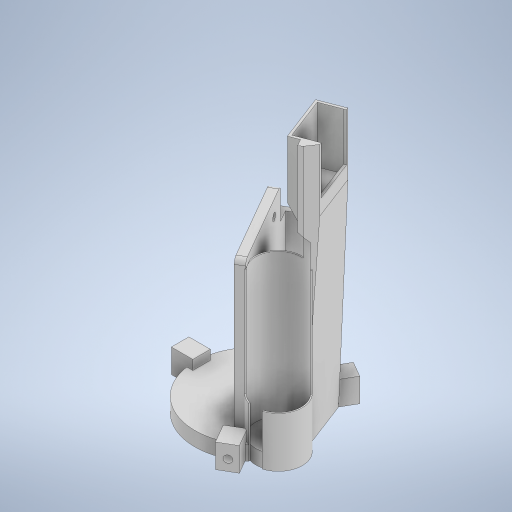
# Autodesk Inventor part: Electronic casing
Saved by Autodesk Inventor 2024 (Build 280153000, 153)
## iProperties
Created: 2024-03-27
Part Number: Electronic casing
Material: Generic
Document SubType Name: Modeling
Designer: auror
Density: 1 g/cm^3
Appearance: Default
Author: auror
Autodesk Inventor part; units mm, degrees
ref_plane "YZ Plane" through (0, 0, 0) normal (1, 0, 0) x (0, 1, 0)
ref_plane "XZ Plane" through (0, 0, 0) normal (0, 1, 0) x (-1, 0, 0)
ref_plane "XY Plane" through (0, 0, 0) normal (0, 0, 1) x (1, 0, 0)
sketch "Sketch9" plane through (0, 0, 0) normal (0, 1, 0) x (-1, 0, 0)
  line L0 (37.6236, 0) -> (-39.3749, 0) construction
  line L1 (0, 0) -> (-26.8726, 46.5447) construction
  line L2 (0, 0) -> (-26.275, -45.5096) construction
  line L3 (31.2294, 3.6686) -> (31.2294, -3.6686)
  line L4 (31.2294, 3.6686) -> (24.7294, 3.6686)
  line L5 (31.2294, -3.6686) -> (24.7294, -3.6686)
  line L6 (0, 0) -> (-18.4784, 42.9064) construction
  line L7 (0, 0) -> (-25.1787, 33.7798) construction
  line L8 (0, 0) -> (31.2294, 3.6686) construction
  line L9 (-12.4376, 28.8797) -> (-18.7918, 25.2111)
  line L10 (-12.4376, 28.8797) -> (-9.1876, 23.2506)
  line L11 (-18.7918, 25.2111) -> (-15.5418, 19.582)
  line L12 (0, 0) -> (-18.2948, -42.48) construction
  line L13 (-18.2948, -42.48) -> (0, 0) construction
  line L14 (0, 0) -> (-26.6993, -35.8199) construction
  line L15 (-18.7918, -25.2111) -> (-12.4376, -28.8797)
  line L16 (-18.7918, -25.2111) -> (-15.5418, -19.582)
  line L17 (-12.4376, -28.8797) -> (-9.1876, -23.2506)
  arc A0 (-15.5418, 19.582) -> (-15.5418, -19.582) centre (0, 0) ccw
  arc A1 (-9.1876, -23.2506) -> (24.7294, -3.6686) centre (0, 0) ccw
  arc A2 (24.7294, 3.6686) -> (-9.1876, 23.2506) centre (0, 0) ccw
  line L18 (0, 0) -> (31.2294, -3.6686) construction
  dimension "d131" = 120
  dimension "d132" = 120
  dimension "d136" = 6.7
  dimension "d137" = 6.7
  dimension "d139" = 6.7
  dimension "d140" = 6.7
  dimension "d220" = 6.5
  dimension "d221" = 6.5
  dimension "d222" = 25
  dimension "d223" = 25
  dimension "d224" = 25
  dimension "d225" = 6.5
  dimension "d227" = 6.5
  dimension "d228" = 6.5
  dimension "d236" = 6.7
  dimension "d237" = 6.7
  constraints: 38 end point, 6 point on circle, 4 perpendicular, 4 point on line, 3 centre point, 3 horizontal, 2 coincident, 1 vertical
  measures "d131" angle of L2 L0
  measures "d132" angle of L1 L0
  measures "d136" angle of L1 L6
  measures "d137" angle of L7 L1
  measures "d139" angle of L2 L12
  measures "d140" angle of L2 L14
  measures "d220" distance of L15.end L17.end
  measures "d221" distance of L9.end L11.end
  measures "d222" radius of A0
  measures "d223" radius of A1
  measures "d224" radius of A2
  measures "d225" distance of L3.end L5.end
  measures "d227" distance of L9.start L10.end
  measures "d228" distance of L15.start L16.end
  measures "d236" angle of L0 L8
  measures "d237" angle of L18 L0
extrude "Extrusion4" add sketch "Sketch9" along normal blind 6
sketch "Sketch10" plane through (18.7918, 0, 25.2111) normal (0.5, 0, 0.8660254) x (0.8660254, 0, -0.5)
  line L0 (0, 0) -> (0, 6) projected
  line L1 (-7.3372, 0) -> (0, 0) projected
  point P0 (-3.6686, 0)
  point P1 (-3.5, 4.5)
  point P2 (0, 3)
  dimension "d143" = 3.5
  dimension "d144" = 4.5
  constraints: 1 midpoint
  measures "d143" horizontal distance of point (0, 3) point (-3.5, 4.5)
  measures "d144" distance from line of L1 point (-3.5, 4.5)
hole "Hole5" at (15.7607, 4.5, 26.9611) direction (-0.5, 0, -0.8660254) diameter 3 depth 8 tip angle 118 counterbore diameter 4 counterbore depth 0
sketch "Sketch11" plane through (12.4376, 0, -28.8797) normal (0.5, 0, -0.8660254) x (-0.8660254, 0, -0.5)
  line L0 (-7.3372, 0) -> (0, 0) projected
  point P0 (-3.6686, 0)
  point P1 (-3.5001, 4.5)
  dimension "d152" = 4.5
  measures "d152" distance from line of L0 point (-3.5, 4.5)
hole "Hole6" at (15.4688, 4.5, -27.1297) direction (-0.5, 0, 0.8660254) diameter 3 depth 8 tip angle 118 counterbore diameter 4 counterbore depth 0
sketch "Sketch12" plane through (-31.2294, 0, -3.6686) normal (-1, 0, 0) x (0, 0, 1)
  line L0 (0, 0) -> (7.3372, 0) projected
  point P0 (3.6686, 0)
  point P1 (3.5, 4.5)
  dimension "d160" = 4.5
  measures "d160" distance from line of L0 point (3.5, 4.5)
hole "Hole7" at (-31.2294, 4.5, -0.1686) direction (1, 0, 0) diameter 3 depth 8 tip angle 118 counterbore diameter 4 counterbore depth 0
sketch "Sketch13" plane through (0, 6, 0) normal (0, 1, 0) x (1, 0, 0)
  line L0 (0, -31.2314) -> (0, 39.2316) construction
  line L1 (11.4285, -21.7947) -> (-13.356, 21.1333) construction
  arc A0 (9.1876, 23.2506) -> (-24.7294, 3.6686) centre (0, 0) ccw construction
  line L2 (8.9539, -17.5087) -> (11.985, -15.7587)
  line L3 (8.9539, -17.5087) -> (-11.0461, 17.1324)
  line L4 (-11.0461, 17.1324) -> (-8.015, 18.8824)
  line L5 (-8.015, 18.8824) -> (11.985, -15.7587)
  dimension "d168" = -30
  dimension "d169" = 1
  dimension "d176" = 40
  dimension "d178" = 3.5
  dimension "d238" = 3.5
  constraints: 12 end point, 2 perpendicular, 2 point on line, 1 collinear, 1 point on circle, 1 vertical
  measures "d168" angle of L0 L1
  measures "d169" distance from line of A0.centre L1
  measures "d176" distance of L3.end L2.start
  measures "d178" distance of L2.start L2.end
  measures "d238" distance of L3.end L4.end
extrude "Extrusion5" add sketch "Sketch13" along normal blind 63
sketch "Sketch14" plane through (0, 6, 0) normal (0, 1, 0) x (1, 0, 0)
  line L0 (11.985, -15.7587) -> (-8.015, 18.8824) projected
  line L1 (-8.015, 18.8824) -> (11.985, -15.7587) projected
  line L2 (2.4652, 31.2084) -> (18.9652, 2.6295)
  line L3 (18.9652, 2.6295) -> (18.3869, -0.3601)
  arc A0 (9.1876, 23.2506) -> (-24.7294, 3.6686) centre (0, 0) ccw projected
  line L4 (-10.7323, 23.5889) -> (0.7369, 30.2107)
  line L5 (0.7369, 30.2107) -> (17.2354, 1.6345)
  line L6 (2.4652, 31.2084) -> (-0.476, 31.9965)
  line L7 (-0.476, 31.9965) -> (-11.8088, 25.4535)
  circle A1 centre (0, 0) radius 32 construction
  line L8 (-10.7323, 23.5889) -> (-8.015, 18.8824)
  line L9 (17.2354, 1.6345) -> (18.3869, -0.3601)
  line L10 (-11.0461, 17.1324) -> (-8.015, 18.8824) projected
  line L11 (-11.0461, 17.1324) -> (-14.8399, 23.7035)
  line L12 (-14.8399, 23.7035) -> (-11.8088, 25.4535)
  line L13 (-11.0461, 17.1324) -> (8.9539, -17.5087) projected
  point P0 (1.985, 1.5618)
  point P1 (-7.7145, 18.3619)
  point P2 (-7.3415, 17.7158)
  point P3 (-10.514, 23.2107)
  dimension "d369" = 64
  dimension "d306" = 33
  dimension "d311" = 1.9956
  dimension "d314" = 3.045
  dimension "d315" = 135
  dimension "d316" = 3.045
  dimension "d317" = 2.153
  constraints: 20 end point, 3 collinear, 2 perpendicular, 2 point on line, 1 coincident, 1 midpoint, 1 parallel, 3 other
  measures "d306" distance of L2.start L2.end
  measures "d311" distance between parallel lines of L5 L2
  measures "d314" distance of L2.end L3.end
  measures "d315" angle of L6 L7
  measures "d316" distance of L2.start L6.end
  measures "d317" distance between parallel lines of L4 L7
extrude "Extrusion6" add sketch "Sketch14" along normal blind 50 contours L2 A0 L5 L4 L8 L11 L12 L7 L6 | L2 L3 L9 L5 A0 | L8 L10 L11 A0
sketch "Sketch15" plane through (8.9539, 6, 17.5087) normal (-0.8660254, 0, 0.5) x (0.5, 0, 0.8660254)
  line L0 (-40, 63) -> (0, 63) projected
  line L1 (-40, 0) -> (-40, 63) projected
  point P0 (-19.6399, -6)
  point P1 (-32.5, 56.6)
  point P2 (-7.5, 56.6)
  point P3 (-7.5, 11.4)
  point P4 (-32.5, 11.4)
  dimension "d201" = 0
  dimension "d202" = 25
  dimension "d203" = 0
  dimension "d204" = 45.2
  dimension "d205" = 0
  dimension "d206" = 25
  dimension "d209" = 6.4
  dimension "d210" = 7.5
  measures "d201" vertical distance of point (-7.5, 56.6) point (-32.5, 56.6)
  measures "d202" distance of point (-7.5, 56.6) point (-32.5, 56.6)
  measures "d203" horizontal distance of point (-7.5, 11.4) point (-7.5, 56.6)
  measures "d204" distance of point (-7.5, 56.6) point (-7.5, 11.4)
  measures "d205" vertical distance of point (-32.5, 11.4) point (-7.5, 11.4)
  measures "d206" distance of point (-7.5, 11.4) point (-32.5, 11.4)
  measures "d209" distance from line of L0 point (-32.5, 56.6)
  measures "d210" distance from line of L1 point (-32.5, 56.6)
hole "Hole8" at (-7.2961, 62.6, -10.6372) at (5.2039, 62.6, 11.0135) at (5.2039, 17.4, 11.0135) at (-7.2961, 17.4, -10.6372) direction (0.8660254, 0, -0.5) diameter 3 depth 15 tip angle 118 counterbore diameter 4 counterbore depth 0
fillet "Fillet3" radius 2 1 edges at (-9.5305, 69, -18.0074)
fillet "Fillet4" radius 2 1 edges at (10.4695, 69, 16.6337)
sketch "Sketch16" plane through (0, 6, 0) normal (0, 1, 0) x (1, 0, 0)
  line L0 (12.4376, -28.8797) -> (18.7918, -25.2111)
  line L1 (12.4376, -28.8797) -> (7.9376, -21.0855)
  line L2 (7.9376, -21.0855) -> (14.2918, -17.4169)
  line L3 (14.2918, -17.4169) -> (18.7918, -25.2111)
  line L4 (18.7918, -25.2111) -> (15.5418, -19.582) projected
  point P0 (0, 0)
  dimension "d231" = 180
  dimension "d232" = 0
  dimension "d240" = 9
  constraints: 8 end point, 2 perpendicular
  measures "d231" angle of L4 L3
  measures "d232" distance of L0.end L3.end
  measures "d240" distance of L0.start L1.end
extrude "Extrusion7" add sketch "Sketch16" along normal blind 4
pattern_circular "Circular Pattern1" count 3 over 360 about axis through (0, -10, 0) along (0, 1, 0) of "Extrusion7"
sketch "Sketch17" plane through (0, 6, 0) normal (0, 1, 0) x (1, 0, 0)
  arc A0 (15.5418, -19.582) -> (15.5418, 19.582) centre (0, 0) ccw projected
  line L0 (15.5418, 19.582) -> (24.6527, -4.1527)
  arc A1 (24.6527, -4.1527) -> (15.5418, 19.582) centre (0, 0) ccw
  line L1 (39.1744, 0) -> (-46.6954, 0) construction
  dimension "d244" = 69
  constraints: 4 end point, 3 point on circle, 1 centre point, 1 coincident, 1 horizontal
  measures "d244" angle of L1 L0
extrude "Extrusion8" cut sketch "Sketch17" against normal through all
sketch "Sketch18" plane through (0, 6, 0) normal (0, 1, 0) x (1, 0, 0)
  line L0 (24.6527, -4.1527) -> (15.5418, 19.582) projected
  line L1 (23.2254, -5.2276) -> (6.6704, 23.2443) projected
  line L2 (21.9165, -2.9764) -> (8.8008, 19.5803)
  line L3 (15.5418, 19.582) -> (18.7918, 25.2111) projected
  line L4 (8.8008, 19.5803) -> (6.6704, 23.2443)
  line L5 (15.5418, 19.582) -> (14.2918, 17.4169) projected
  line L6 (15.5418, 19.582) -> (24.6527, -4.1527)
  line L7 (23.2254, -5.2276) -> (24.6527, -4.1527)
  line L8 (23.2254, -5.2276) -> (21.9165, -2.9764)
  line L9 (15.5418, 19.582) -> (7.9196, 21.0959)
  point P0 (0, 0)
  point P1 (9.6696, 20.0855)
  constraints: 12 end point, 4 point on line, 3 collinear
extrude "Extrusion9" add sketch "Sketch18" along normal blind 105
sketch "Sketch19" plane through (24.6527, 0, 4.1527) normal (0.9335804, 0, -0.3583679) x (-0.3583679, 0, -0.9335804)
  line L0 (0, 6) -> (25.4233, 6) projected
  line L1 (2.75, 111) -> (23.25, 111)
  line L2 (23.25, 111) -> (23.25, 80)
  line L3 (2.75, 80) -> (2.75, 111)
  line L4 (2.4233, 6) -> (2.4233, 111) projected
  line L5 (0, 6) -> (0, 111) projected
  line L6 (0, 111) -> (25.4233, 111) projected
  line L7 (23.25, 80) -> (2.75, 80)
  line L8 (25.4233, 0) -> (0, 0) projected
  point P0 (12.7116, 0)
  point P1 (13, 0)
  dimension "d251" = 20.5
  dimension "d254" = 10.25
  dimension "d267" = 13
  dimension "d290" = 31
  constraints: 8 end point, 2 parallel, 1 horizontal, 1 perpendicular, 1 point on line
  measures "d251" distance of L2.end L3.start
  measures "d254" distance from line of L3 point (13, 0)
  measures "d267" distance from line of L5 point (13, 0)
  measures "d290" distance of L1.end L2.end
extrude "Extrusion10" add sketch "Sketch19" along normal blind 4 and the other way blind 6.5 contours L1 L2 L7 L3
sketch "Sketch22" plane through (0, 111, 0) normal (0, 1, 0) x (1, 0, 0)
  line L0 (18.1741, -2.6228) -> (26.1095, 0.4233)
  line L1 (26.1095, 0.4233) -> (19.4797, 17.6945)
  line L2 (19.4797, 17.6945) -> (11.5443, 14.6484)
  line L3 (11.5443, 14.6484) -> (18.1741, -2.6228)
  line L4 (23.6672, -1.5854) -> (27.4015, -0.1519) projected
  line L5 (16.3206, 17.553) -> (20.0549, 18.9865) projected
  line L6 (17.5989, -3.9148) -> (10.2524, 15.2236) projected
  line L7 (20.0549, 18.9865) -> (27.4015, -0.1519) projected
  line L8 (17.5989, -3.9148) -> (21.5747, -2.3886) projected
  point P0 (0, 0)
  dimension "d270" = 18.5
  dimension "d271" = 8.5
  dimension "d272" = 1
  dimension "d273" = 1
  constraints: 8 end point, 4 parallel, 1 perpendicular
  measures "d270" distance of L0.end L1.end
  measures "d271" distance of L1.end L2.end
  measures "d272" distance between parallel lines of L3 L6
  measures "d273" distance between parallel lines of L8 L0
extrude "Extrusion13" cut sketch "Sketch22" against normal blind 23.5
sketch "Sketch23" plane through (0, 111, 0) normal (0, 1, 0) x (1, 0, 0)
  line L0 (19.4797, 17.6945) -> (26.1095, 0.4233) projected
  line L1 (26.1095, 0.4233) -> (27.0431, 0.7817)
  line L2 (20.0549, 18.9865) -> (27.4015, -0.1519) projected
  line L3 (19.5009, 17.6394) -> (20.4345, 17.9978)
  line L4 (20.4345, 17.9978) -> (27.0431, 0.7817)
  line L5 (26.1095, 0.4233) -> (19.5009, 17.6394)
  line L6 (19.4797, 17.6945) -> (26.1095, 0.4233) projected
  point P0 (0, 0)
  constraints: 8 end point, 3 perpendicular, 1 parallel, 1 point on line
extrude "Extrusion14" cut sketch "Sketch23" against normal blind 20
chamfer "Chamfer4" distance 4 angle 60 1 edges at (13.9256, 80, -5.6544) measured on face at (14.3924, 80, -5.8336)
sketch "Sketch24" plane through (0, 111, 0) normal (0, 1, 0) x (1, 0, 0)
  arc A0 (15.5418, -19.582) -> (24.6527, -4.1527) centre (0, 0) ccw projected
  line L0 (24.6527, -4.1527) -> (23.6656, -1.5813)
  line L1 (15.5418, 19.582) -> (24.6527, -4.1527) projected
  line L2 (23.6672, -1.5854) -> (27.4015, -0.1519) projected
  line L3 (27.4015, -0.1519) -> (24.6527, -4.1527)
  line L4 (16.3213, 17.5513) -> (15.5418, 19.582)
  line L5 (16.3206, 17.553) -> (20.0549, 18.9865) projected
  line L6 (15.5418, 19.582) -> (20.0549, 18.9865)
  line L7 (20.0549, 18.9865) -> (16.3206, 17.553)
  constraints: 10 end point, 2 point on line, 1 collinear
extrude "Extrusion15" add sketch "Sketch24" against normal blind 111
sketch "Sketch26" plane through (16.3206, 80, -17.553) normal (0, -1, 0) x (0.9335804, 0, -0.3583679)
  line L0 (4, 20.5) -> (0, 20.5) projected
  line L1 (0, 20.5) -> (4, 20.5)
  line L2 (4, 20.5) -> (4, 0)
  line L3 (4, 0) -> (0, 0)
  line L4 (0, 0) -> (0, 20.5)
  point P0 (-21.5271, 10.5384)
  point P1 (-2.5, 20.5)
  constraints: 8 end point, 2 parallel, 1 horizontal, 1 perpendicular
extrude "Extrusion16" add sketch "Sketch26" along normal blind 80
chamfer "Chamfer6" distance 85 angle 2.694 1 edges at (23.7282, 0, -9.4173) measured on face at (23.7282, 0.5, -9.4173)
sketch "Sketch27" plane through (0, 111, 0) normal (0, 1, 0) x (1, 0, 0)
  line L0 (15.5419, 19.5819) -> (20.0549, 18.9865) projected
  line L1 (6.6704, 23.2443) -> (15.5419, 19.5819)
  line L2 (20.0549, 18.9865) -> (27.4015, -0.1519) projected
  line L3 (15.5419, 19.5819) -> (20.0549, 18.9865)
  line L4 (10.2524, 15.2236) -> (11.1367, 15.5631) projected
  line L5 (20.0549, 18.9865) -> (11.1367, 15.5631)
  line L6 (11.1367, 15.5631) -> (6.6704, 23.2443)
  point P0 (0, 0)
  constraints: 8 end point, 1 collinear
extrude "Extrusion17" cut sketch "Sketch27" against normal blind 17
fillet "Face Fillet1" radius 1 1 edges at (15.5958, 94, -17.2748)
sketch "Sketch38" plane through (0, 6, 0) normal (0, 1, 0) x (1, 0, 0)
  line L0 (2.4652, 31.2084) -> (-0.476, 31.9965) projected
  line L1 (-0.476, 31.9965) -> (-11.5905, 25.0753)
  line L2 (8.3534, 21.0097) -> (2.4652, 31.2084) projected
  line L3 (-0.476, 31.9965) -> (2.4652, 31.2084)
  arc A0 (9.1876, 23.2506) -> (-24.7294, 3.6686) centre (0, 0) ccw projected
  line L4 (2.4652, 31.2084) -> (6.5546, 24.1255)
  arc A1 (6.2227, 24.2132) -> (14.6024, -20.2921) centre (0, 0) ccw
  line L5 (8.9539, -17.5087) -> (-13.356, 21.1333) projected
  line L6 (-13.356, 21.1333) -> (-14.6216, 23.3253)
  line L7 (-14.6216, 23.3253) -> (-11.5905, 25.0753)
  line L8 (-13.356, 21.1333) -> (-6.4888, 10.7302)
  line L9 (-6.4888, 10.7302) -> (6.2227, 24.2132)
  point P0 (3.9242, 24.6901)
  point P1 (6.5546, 24.1255)
  constraints: 14 end point, 2 point on circle, 1 centre point, 1 coincident, 1 collinear, 1 perpendicular
extrude "Extrusion24" add sketch "Sketch38" against normal blind 6 contours L2 A0 L6 L7 L1 L0
sketch "Sketch39" plane through (0, 6, 0) normal (0, 1, 0) x (1, 0, 0)
  circle A0 centre (19.2133, -9.2784) radius 9.5
  line L0 (10.985, -14.0266) -> (-7.015, 17.1503) projected
  circle A1 centre (0, 0) radius 33 construction
  circle A2 centre (19.2133, -9.2784) radius 10
  line L1 (17.2444, 1.1319) -> (5.986, -5.3681) construction
  dimension "d372" = 19
  dimension "d373" = 66
  dimension "d374" = 20
  constraints: 3 centre point, 2 coincident, 2 tangent
  measures "d372" diameter of A0
  measures "d373" diameter of A1
  measures "d374" diameter of A2
extrude "Extrusion25" add sketch "Sketch39" along normal blind 60
sketch "Sketch40" plane through (0, 66, 0) normal (0, 1, 0) x (1, 0, 0)
  arc A0 (18.0896, 0.1549) -> (16.8402, -18.4772) centre (19.2133, -9.2784) ccw projected
  arc A1 (16.8402, -18.4772) -> (23.7106, -0.9103) centre (19.2133, -9.2784) ccw projected
  arc A2 (12.3698, -15.8675) -> (26.0568, -2.6893) centre (19.2133, -9.2784) ccw
  arc A3 (11.7266, -15.9078) -> (13.8117, -17.694) centre (19.2133, -9.2784) ccw projected
  arc A4 (16.3953, -18.8731) -> (23.4448, -0.2178) centre (19.2133, -9.2784) ccw projected
  arc A5 (12.0096, -16.2143) -> (26.417, -2.3425) centre (19.2133, -9.2784) ccw
  line L0 (12.0096, -16.2143) -> (12.3698, -15.8675)
  line L1 (26.417, -2.3425) -> (26.0568, -2.6893)
  line L2 (12.0096, -16.2143) -> (26.417, -2.3425) construction
  point P0 (0, 0)
  point P1 (13.8117, -17.694)
  constraints: 8 point on circle, 6 end point, 2 centre point, 2 point on line, 1 midpoint
extrude "Extrusion26" cut sketch "Sketch40" against normal blind 45
sketch "Sketch42" plane through (0, 6, 0) normal (0, 1, 0) x (1, 0, 0)
  circle A0 centre (19.2133, -9.2784) radius 9.5
  arc A1 (12.3698, -15.8675) -> (26.0568, -2.6893) centre (19.2133, -9.2784) ccw projected
  point P0 (0, 0)
  dimension "d379" = 19
  constraints: 1 centre point, 1 concentric
  measures "d379" diameter of A0
extrude "Extrusion27" cut sketch "Sketch42" along normal blind 73.5
chamfer "Chamfer10" distance 3.7 angle 45 1 edges at (23.1758, 79.5, 0.6442)
sketch "Sketch43" plane through (0, 6, 0) normal (0, 1, 0) x (1, 0, 0)
  circle A0 centre (19.2133, -9.2784) radius 10
  arc A1 (12.0096, -16.2143) -> (26.417, -2.3425) centre (19.2133, -9.2784) ccw projected
  point P0 (0, 0)
  dimension "d385" = 20
  constraints: 1 centre point, 1 concentric
  measures "d385" diameter of A0
extrude "Extrusion28" add sketch "Sketch43" against normal blind 6
sketch "Sketch44" plane through (0, 21, 0) normal (0, 1, 0) x (1, 0, 0)
  arc A0 (16.3953, -18.8731) -> (23.0804, -0.0563) centre (19.2133, -9.2784) ccw projected
  arc A1 (16.3953, -18.8731) -> (22.0312, -18.8731) centre (19.2133, -9.2784) ccw
  circle A2 centre (19.2133, -9.2784) radius 9.5 projected
  arc A3 (16.3953, -18.3508) -> (21.8548, -18.4037) centre (19.2133, -9.2784) ccw
  line L0 (16.3953, -18.3508) -> (16.3953, -18.8731)
  line L1 (21.8548, -18.4037) -> (22.0312, -18.8731)
  point P0 (0, 0)
  point P1 (16.3953, -18.8731)
  constraints: 7 point on circle, 4 end point, 2 centre point
extrude "Extrusion29" cut sketch "Sketch44" against normal blind 21 contours L0 A2 L1 A0
sketch "Sketch45" plane through (0, 6, 0) normal (0, 1, 0) x (1, 0, 0)
  line L0 (18.8883, 2.2316) -> (7.9196, 21.0959) projected
  arc A0 (19.7754, 0.7058) -> (9.4248, -11.3242) centre (19.2133, -9.2784) ccw projected
  line L1 (18.8883, 2.2316) -> (19.7754, 0.7058)
  line L2 (19.7754, 0.7058) -> (18.8883, 2.2316)
  line L3 (17.2053, 1.6867) -> (4.316, -5.755)
  line L4 (0.7369, 30.2107) -> (17.8188, 0.6239) projected
  line L5 (10.985, -14.0266) -> (7.9539, -15.7766) projected
  arc A1 (20.5511, 0.127) -> (10.985, -14.0266) centre (19.2133, -9.2784) ccw
  line L6 (5.736, -4.9351) -> (10.985, -14.0266)
  line L7 (-10.0461, 15.4003) -> (7.9539, -15.7766) projected
  line L8 (10.985, -14.0266) -> (-7.015, 17.1503) projected
  line L9 (20.7594, -0.9865) -> (11.1367, 15.5631) projected
  line L10 (17.2053, 1.6867) -> (18.6998, 2.5557)
  point P0 (0, 0)
  point P1 (13.3835, -1.1535)
  point P2 (11.1367, 15.5631)
  dimension "d392" = 0.5
  constraints: 10 end point, 2 perpendicular, 2 point on circle, 2 point on line, 1 centre point, 1 coincident, 1 collinear, 1 parallel, 2 other
  measures "d392" distance edge to line of A0 L3
extrude "Extrusion30" add sketch "Sketch45" along normal blind 50 contours L1 A0 L4 L10 L0 | L4 A0 L6 L3
body "Solid2"
